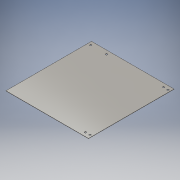
# Autodesk Inventor part: MC Part2
Saved by Autodesk Inventor 2016 (Build 200138000, 138)
## iProperties
Created: 2017-10-17
Part Number: MC Part2
Material: Steel, Mild
Document SubType Name: Sheet Metal
Designer: m207653
Density: 7.85 g/cm^3
Sheet Metal Rule: ms steel
Appearance: Semi-Polished
Flat Pattern Width: 55 cm
Flat Pattern Length: 57 cm
Flat Pattern Area: 3135 cm^2
Sheet Metal Width: 550.000 mm
Sheet Metal Length: 570.000 mm
Sheet Metal Area: 313500.000 mm^2
Author: m207653
Autodesk Inventor part; units mm, degrees
ref_plane "YZ Plane" through (0, 0, 0) normal (1, 0, 0) x (0, 1, 0)
ref_plane "XZ Plane" through (0, 0, 0) normal (0, 1, 0) x (-1, 0, 0)
ref_plane "XY Plane" through (0, 0, 0) normal (0, 0, 1) x (1, 0, 0)
sketch "Sketch1" plane through (0, 0, 0) normal (0, 0, 1) x (1, 0, 0)
  line L0 (0, 1125) -> (0, 1695)
  line L1 (0, 1695) -> (550, 1695)
  line L2 (550, 1695) -> (550, 1125)
  line L3 (550, 1125) -> (0, 1125)
  point P0 (0, 0)
  dimension "d2" = 550
  dimension "d3" = 570
  constraints: 8 end point, 3 perpendicular, 1 vertical
  measures "d2" distance of L0.end L1.end
  measures "d3" distance of L1.end L2.end
extrude "Plate1" add sketch "Sketch1" along normal blind 1.6
sketch "Sketch7" plane through (0, 0, 1.6) normal (0, 0, 1) x (1, 0, 0)
  line L0 (0, 1695) -> (550, 1695) projected
  line L1 (490, 1695) -> (490, 1125)
  line L2 (550, 1125) -> (0, 1125) projected
  line L3 (550, 1695) -> (550, 1125) projected
  circle A0 centre (535, 1670) radius 6
  circle A1 centre (505, 1670) radius 6
  circle A2 centre (535, 1150) radius 6
  circle A3 centre (505, 1150) radius 6
  point P0 (0, 0)
  point P1 (1.1647, 1695)
  point P2 (150, 1125)
  point P3 (1.1647, 1125)
  dimension "d57" = 60
  dimension "d58" = 12
  dimension "d59" = 12
  dimension "d60" = 15
  dimension "d61" = 15
  dimension "d62" = 25
  dimension "d63" = 25
  dimension "d64" = 12
  dimension "d65" = 12
  dimension "d66" = 25
  dimension "d67" = 25
  dimension "d75" = 15
  dimension "d76" = 15
  constraints: 4 centre point, 2 end point, 2 point on line, 1 vertical
  measures "d57" distance between parallel lines of L1 L3
  measures "d58" diameter of A0
  measures "d59" diameter of A1
  measures "d60" distance from line of L3 A0.centre
  measures "d61" distance from line of L1 A1.centre
  measures "d62" distance from line of L0 A0.centre
  measures "d63" distance from line of L0 A1.centre
  measures "d64" diameter of A2
  measures "d65" diameter of A3
  measures "d66" distance from line of L2 A2.centre
  measures "d67" distance from line of L2 A3.centre
  measures "d75" distance from line of L1 A3.centre
  measures "d76" distance from line of A2.centre L3
hole "Hole3" at (535, 1670, 1.6) at (505, 1670, 1.6) at (535, 1150, 1.6) at (505, 1150, 1.6) direction (0, 0, -1) diameter 12 end through all
sketch "Sketch8" plane through (0, 0, 1.6) normal (0, 0, 1) x (1, 0, 0)
  line L0 (0, 1695) -> (0, 1125) projected
  line L1 (0, 1695) -> (145, 1695)
  line L2 (550, 1695) -> (0, 1695) projected
  line L3 (145, 1695) -> (145, 1125)
  line L4 (0, 1125) -> (550, 1125) projected
  circle A0 centre (125, 1670) radius 6
  circle A1 centre (20, 1670) radius 6
  point P0 (0, 0)
  dimension "d79" = 145
  dimension "d80" = 12
  dimension "d81" = 25
  dimension "d82" = 20
  dimension "d83" = 12
  dimension "d84" = 20
  constraints: 4 end point, 2 centre point, 2 point on line, 1 perpendicular
  measures "d79" distance of L0.start L1.end
  measures "d80" diameter of A0
  measures "d81" distance from line of L1 A0.centre
  measures "d82" distance from line of L3 A0.centre
  measures "d83" diameter of A1
  measures "d84" distance from line of L0 A1.centre
hole "Hole4" at (125, 1670, 1.6) at (20, 1670, 1.6) direction (0, 0, -1) diameter 12 end through all
equation "\"d73\" = Thickness"
equation "\"d90\" = Thickness"
equation "\"BendRadius\" = Thickness"
equation "\"BendReliefWidth\" = Thickness"
equation "\"BendReliefDepth\" = 0.5 * Thickness"
equation "\"CornerReliefSize\" = 4 * Thickness"
equation "\"MinimumRemnant\" = 2 * Thickness"
equation "\"TransitionRadius\" = BendRadius"
equation "\"JacobiRadiusSize\" = BendRadius"
equation "\"GapSize\" = Thickness"
equation "\"d4\" = BendRadius"
equation "\"Thickness\" = 1.6"
body "Solid1"
